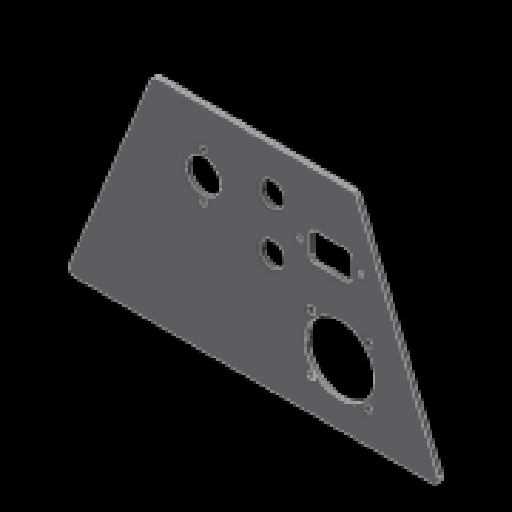
# Autodesk Inventor part: BreakerMount
Saved by Autodesk Inventor 2025.2 (Build 292293000, 293)
## iProperties
Created: 2025-11-18
Part Number: BreakerMount
Material: Generic
Document SubType Name: Sheet Metal
Designer: valer
Density: 1 g/cm^3
Sheet Metal Rule: Default
Appearance: Default
Author: valer
Autodesk Inventor part; units mm, degrees
ref_plane "YZ Plane" through (0, 0, 0) normal (1, 0, 0) x (0, 1, 0)
ref_plane "XZ Plane" through (0, 0, 0) normal (0, 1, 0) x (-1, 0, 0)
ref_plane "XY Plane" through (0, 0, 0) normal (0, 0, 1) x (1, 0, 0)
sketch "Base" plane through (0, 0, 0) normal (0, 0, 1) x (1, 0, 0)
  line L0 (0, 0) -> (70.3402, 0)
  line L1 (70.3402, 0) -> (142.1613, -140)
  line L2 (142.1613, -140) -> (0, -140)
  line L3 (0, -140) -> (0, 0) construction
  line L4 (0, 0) -> (-70.3402, 0)
  line L5 (-70.3402, 0) -> (-142.1613, -140)
  line L6 (-142.1613, -140) -> (0, -140)
  line L7 (-63.3831, 22.3248) -> (-182.4251, -209.7225) construction
  dimension "d1" = 140
  dimension "d3" = 4
  measures "d1" distance between parallel lines of L6 L4
  measures "d3" distance between parallel lines of L7 L5
extrude "Plate1" add sketch "Base" along normal blind 3
fillet "FilletsFeature" radius 6 4 edges at (-70.3402, 0, 1.5) (70.3402, 0, 1.5) (142.1613, -140, 1.5) (-142.1613, -140, 1.5)
sketch "MatchProduction" plane through (0, 0, 3) normal (0, 0, 1) x (1, 0, 0)
  line L0 (0, -169.9469) -> (0, 29.2004) construction
  line L1 (-66.6748, 0) -> (66.6748, 0) projected
  line L2 (66.6748, 0) -> (123.2385, -140)
  line L3 (132.3398, -140) -> (-132.3398, -140) projected
  arc A0 (72.0133, -3.2613) -> (66.6748, 0) centre (66.6748, -6) ccw projected
  line L4 (72.0133, -3.2613) -> (137.6783, -131.2613) projected
  arc A1 (132.3398, -140) -> (137.6783, -131.2613) centre (132.3398, -134) ccw projected
  arc A2 (-137.6783, -131.2613) -> (-132.3398, -140) centre (-132.3398, -134) ccw projected
  line L5 (-137.6783, -131.2613) -> (-72.0133, -3.2613) projected
  arc A3 (-66.6748, 0) -> (-72.0133, -3.2613) centre (-66.6748, -6) ccw projected
  line L6 (-66.6748, 0) -> (-123.2385, -140)
  point P0 (0, 0)
  point P1 (-123.2385, -140)
  dimension "d13" = 68
  constraints: 4 end point, 1 point on line, 1 symmetric about line
  measures "d13" angle of L3 L2
extrude "MatchProductionFeature" cut sketch "MatchProduction" against normal blind 3 contours L6 L3 A2 L5 A3 | A0 L4 A1 L3 L2
fillet "OutsideFilletsFeature" radius 4 4 edges at (-123.2385, -140, 1.5) (123.2385, -140, 1.5) (66.6748, 0, 1.5) (-66.6748, 0, 1.5)
sketch "PanelControls" plane through (0, 0, 0) normal (0, 0, -1) x (-1, 0, 0)
  circle A0 centre (33, -55.3581) radius 2 projected
  circle A1 centre (33, -25.3581) radius 2 projected
  circle A2 centre (-12, -62.1443) radius 8 projected
  circle A3 centre (-12, -28.2391) radius 8 projected
  circle A4 centre (-37.8, -81.5) radius 2.5 projected
  circle A5 centre (-37.8, -118.5) radius 2.5 projected
  circle A6 centre (-74.8, -118.5) radius 2.5 projected
  circle A7 centre (-74.8, -81.5) radius 2.5 projected
  circle A8 centre (-30.3, -44.3793) radius 1.65 projected
  circle A9 centre (-70.3, -44.3793) radius 1.65 projected
  circle A10 centre (-56.3, -100) radius 22.5 projected
  arc A11 (33, -51.4831) -> (33, -29.2331) centre (33, -40.3581) ccw projected
  line L0 (-39.75, -53.7293) -> (-60.85, -53.7293) projected
  arc A12 (-39.75, -53.7293) -> (-36.75, -50.7293) centre (-39.75, -50.7293) ccw projected
  line L1 (-36.75, -38.0293) -> (-36.75, -50.7293) projected
  arc A13 (-36.75, -38.0293) -> (-39.75, -35.0293) centre (-39.75, -38.0293) ccw projected
  line L2 (-60.85, -35.0293) -> (-39.75, -35.0293) projected
  arc A14 (-60.85, -35.0293) -> (-63.85, -38.0293) centre (-60.85, -38.0293) ccw projected
  line L3 (-63.85, -50.7293) -> (-63.85, -38.0293) projected
  arc A15 (-63.85, -50.7293) -> (-60.85, -53.7293) centre (-60.85, -50.7293) ccw projected
  arc A16 (33, -51.4831) -> (33, -29.2331) centre (33, -40.3581) ccw projected
  circle A17 centre (33, -40.3581) radius 11.125 projected
  line L4 (80.8, -122.5) -> (80.8, -77.5) construction
  line L5 (80.8, -77.5) -> (26.8, -77.5) construction
  line L6 (26.8, -122.5) -> (80.8, -122.5) construction
  line L7 (26.8, -77.5) -> (26.8, -122.5) construction
  line L8 (0.05, -122.575) -> (26.8, -122.575) construction
  line L9 (26.8, -77.425) -> (0.05, -77.425) construction
  line L10 (-26.8, -122.575) -> (-0.05, -122.575) construction
  line L11 (-0.05, -77.425) -> (-26.8, -77.425) construction
  line L12 (-26.8, -122.575) -> (-26.8, -77.425) construction
  line L13 (26.8, -122.575) -> (80.8, -122.575) construction
  line L14 (80.8, -122.575) -> (80.8, -122.5)
  line L15 (80.8, -77.5) -> (80.8, -77.425)
  line L16 (80.8, -77.425) -> (26.8, -77.425) construction
  line L17 (80.8, -122.575) -> (-26.8, -122.575)
  line L18 (-26.8, -122.575) -> (-26.8, -77.425)
  line L19 (-26.8, -77.425) -> (80.8, -77.425)
  line L20 (80.8, -77.425) -> (80.8, -122.575)
  point P0 (0, 0)
  constraints: 18 end point, 3 perpendicular, 2 collinear, 2 parallel, 1 horizontal, 1 vertical
extrude "PanelControlsFeature" cut sketch "PanelControls" against normal blind 3
sketch "PanelControlsBreathingRoom" plane through (0, 0, 0) normal (0, 0, -1) x (-1, 0, 0)
  circle A0 centre (-70.3, -44.3793) radius 1.65 projected
  circle A1 centre (-74.8, -81.5) radius 2.5 projected
  circle A2 centre (-12, -28.2391) radius 8 projected
  circle A3 centre (33, -55.3581) radius 2 projected
  circle A4 centre (-12, -62.1443) radius 8 projected
  circle A5 centre (-37.8, -81.5) radius 2.5 projected
  arc A6 (-60.85, -35.0293) -> (-63.85, -38.0293) centre (-60.85, -38.0293) ccw projected
  line L0 (-60.85, -35.0293) -> (-39.75, -35.0293) projected
  arc A7 (-36.75, -38.0293) -> (-39.75, -35.0293) centre (-39.75, -38.0293) ccw projected
  line L1 (-36.75, -38.0293) -> (-36.75, -50.7293) projected
  arc A8 (-39.75, -53.7293) -> (-36.75, -50.7293) centre (-39.75, -50.7293) ccw projected
  line L2 (-39.75, -53.7293) -> (-60.85, -53.7293) projected
  arc A9 (-63.85, -50.7293) -> (-60.85, -53.7293) centre (-60.85, -50.7293) ccw projected
  line L3 (-63.85, -50.7293) -> (-63.85, -38.0293) projected
  circle A10 centre (-30.3, -44.3793) radius 1.65 projected
  circle A11 centre (-74.8, -118.5) radius 2.5 projected
  circle A12 centre (33, -40.3581) radius 11.125 projected
  circle A13 centre (33, -25.3581) radius 2 projected
  circle A14 centre (-37.8, -118.5) radius 2.5 projected
  circle A15 centre (-56.3, -100) radius 22.5 projected
  line L4 (80.8, -122.575) -> (-26.8, -122.575) projected
  line L5 (-26.8, -122.575) -> (-26.8, -77.425) projected
  line L6 (-26.8, -77.425) -> (80.8, -77.425) projected
  line L7 (80.8, -77.425) -> (80.8, -122.575) projected
  arc A16 (67.6855, -2.5016) -> (63.9768, 0) centre (63.9768, -4) ccw projected
  line L8 (-63.9768, 0) -> (63.9768, 0) projected
  arc A17 (-63.9768, 0) -> (-67.6855, -2.5016) centre (-63.9768, -4) ccw projected
  line L9 (-67.6855, -2.5016) -> (-121.017, -134.5016) projected
  arc A18 (-121.017, -134.5016) -> (-117.3082, -140) centre (-117.3082, -136) ccw projected
  line L10 (117.3082, -140) -> (-117.3082, -140) projected
  arc A19 (117.3082, -140) -> (121.017, -134.5016) centre (117.3082, -136) ccw projected
  line L11 (121.017, -134.5016) -> (67.6855, -2.5016) projected
  line L12 (-27.05, -122.825) -> (81.05, -122.825)
  line L13 (81.05, -122.825) -> (81.05, -77.175)
  line L14 (81.05, -77.175) -> (-27.05, -77.175)
  line L15 (-27.05, -77.175) -> (-27.05, -122.825)
  circle A20 centre (-56.3, -100) radius 22.75
  circle A21 centre (33, -40.3581) radius 11.375
  circle A22 centre (-12, -62.1443) radius 8.25
  circle A23 centre (-12, -28.2391) radius 8.25
  line L16 (-60.85, -53.9793) -> (-39.75, -53.9793)
  arc A24 (-39.75, -53.9793) -> (-36.5, -50.7293) centre (-39.75, -50.7293) ccw
  line L17 (-36.5, -50.7293) -> (-36.5, -38.0293)
  arc A25 (-36.5, -38.0293) -> (-39.75, -34.7793) centre (-39.75, -38.0293) ccw
  line L18 (-39.75, -34.7793) -> (-60.85, -34.7793)
  arc A26 (-60.85, -34.7793) -> (-64.1, -38.0293) centre (-60.85, -38.0293) ccw
  line L19 (-64.1, -38.0293) -> (-64.1, -50.7293)
  arc A27 (-64.1, -50.7293) -> (-60.85, -53.9793) centre (-60.85, -50.7293) ccw
  point P0 (0, 0)
  dimension "d27" = 0.25
  dimension "d28" = 0.25
  dimension "d29" = 0.25
  dimension "d30" = 0.25
  dimension "d31" = 0.25
  dimension "d32" = 0.25
  constraints: 16 end point, 8 centre point, 8 point on circle, 10 other
  measures "d27" distance between parallel lines of L4 L12
  measures "d28" radial gap between concentric circles of A15 A20
  measures "d29" radial gap between concentric circles of A12 A21
  measures "d30" radial gap between concentric circles of A4 A22
  measures "d31" radial gap between concentric circles of A2 A23
  measures "d32" distance between parallel lines of L2 L16
extrude "PanelControlsBreathingRoomFeature" cut sketch "PanelControlsBreathingRoom" against normal blind 3 contours A4 | L0 A7 L1 A8 L2 A9 L3 A6 | A15 | L15 L14 L13 L12 | A20 | A21 | A22 | A23 | A27 L19 A26 L18 A25 L17 A24 L16
equation "\"d14\" = Thickness"
equation "\"d17\" = Thickness"
equation "\"d33\" = Thickness"
equation "\"d0\" = Thickness"
equation "\"BendRadius\" = Thickness"
equation "\"BendReliefWidth\" = Thickness"
equation "\"BendReliefDepth\" = 0.5 * Thickness"
equation "\"CornerReliefSize\" = 4 * Thickness"
equation "\"MinimumRemnant\" = 2 * Thickness"
equation "\"TransitionRadius\" = BendRadius"
equation "\"JacobiRadiusSize\" = BendRadius"
equation "\"GapSize\" = Thickness"
equation "\"Thickness\" = 3"
body "Solid1"
